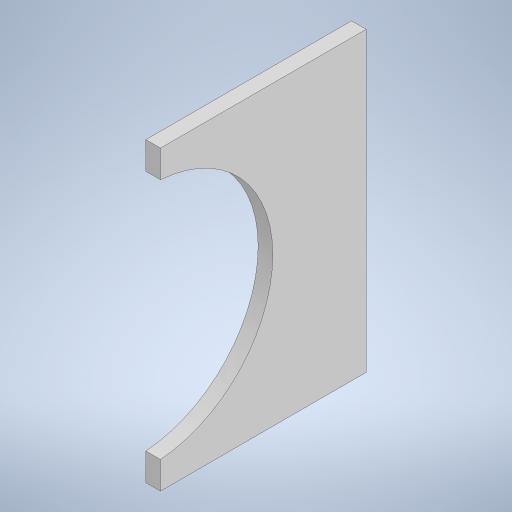
# Autodesk Inventor part: SideSupports
Saved by Autodesk Inventor 2024 (Build 280153000, 153)
## iProperties
Created: 2023-10-07
Part Number: SideSupports
Material: Generic
Document SubType Name: Modeling
Designer: chris
Density: 1 g/cm^3
Appearance: Default
Author: chris
Autodesk Inventor part; units mm, degrees
ref_plane "YZ Plane" through (0, 0, 0) normal (1, 0, 0) x (0, 1, 0)
ref_plane "XZ Plane" through (0, 0, 0) normal (0, 1, 0) x (-1, 0, 0)
ref_plane "XY Plane" through (0, 0, 0) normal (0, 0, 1) x (1, 0, 0)
sketch "Sketch1" plane through (0, 0, 0) normal (1, 0, 0) x (0, 1, 0)
  line L0 (-32.5, 22.5) -> (32.5, 22.5)
  line L1 (32.5, 22.5) -> (32.5, -22.5)
  line L2 (32.5, -22.5) -> (-32.5, -22.5)
  line L3 (-32.5, -22.5) -> (-32.5, 22.5)
  line L4 (-32.5, 22.5) -> (32.5, -22.5) construction
  line L5 (32.5, 22.5) -> (-32.5, -22.5) construction
  arc A0 (-26.5, 22.5) -> (26.5, 22.5) centre (0, 24.5) ccw
  point P0 (0, 0)
  point P1 (0, 22.5)
  dimension "d0" = 45
  dimension "d1" = 65
  dimension "d3" = 6
  dimension "d4" = 6
  dimension "d5" = 2
  constraints: 12 end point, 3 midpoint, 2 parallel, 2 point on circle, 2 point on line, 1 centre point, 1 horizontal, 1 perpendicular
  measures "d0" distance of L0.end L1.end
  measures "d1" distance of L1.end L2.end
  measures "d3" distance from line of L1 A0.end
  measures "d4" distance from line of L3 A0.start
  measures "d5" distance of point (0, 22.5) A0.centre
extrude "Extrusion1" add sketch "Sketch1" along normal blind 3.2 contours L0 A0 L1 L2 L3
body "Solid1"
